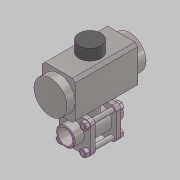
# Autodesk Inventor part: PNEUMATIC BUTT WELD BALL VALVE DN25 304L
Saved by Autodesk Inventor 2017 (Build 210142000, 142)
## iProperties
Category: Plant Design Equipment
Company: Pocket Brewery Belgium
Created: 2017-11-25
Part Number: PNEUMATIC BUTT WELD BALL VALVE DN25 304L
Material: 304L
Document SubType Name: Modeling
Designer: Demarec
Density: 8 g/cm^3
Appearance: Semi-Polished
Description: BELVEN BV3
Author: Marc Crauwels
Title: Valves
Comments: This Valve is generated with the Pocket Brewery Valve App. This software is part of the Pocket Brewery Design Suite.
Autodesk Inventor part; units mm, degrees
ref_plane "YZ Plane" through (0, 0, 0) normal (1, 0, 0) x (0, 1, 0)
ref_plane "XZ Plane" through (0, 0, 0) normal (0, 1, 0) x (-1, 0, 0)
sketch "Sketch3" plane through (0, 0, 0) normal (0, 1, 0) x (-1, 0, 0)
  line L0 (-6.4482, 15.5674) -> (6.4482, 15.5674)
  line L1 (6.4482, 15.5674) -> (15.5674, 6.4482)
  line L2 (15.5674, 6.4482) -> (15.5674, -6.4482)
  line L3 (15.5674, -6.4482) -> (6.4482, -15.5674)
  line L4 (6.4482, -15.5674) -> (-6.4482, -15.5674)
  line L5 (-6.4482, -15.5674) -> (-15.5674, -6.4482)
  line L6 (-15.5674, -6.4482) -> (-15.5674, 6.4482)
  line L7 (-15.5674, 6.4482) -> (-6.4482, 15.5674)
  circle A0 centre (0, 0) radius 16.85
  line L8 (21.375, -28.5) -> (-21.375, -28.5)
  line L9 (-28.5, -21.375) -> (-28.5, 21.375)
  line L10 (-21.375, 28.5) -> (21.375, 28.5)
  line L11 (28.5, 21.375) -> (28.5, -21.375)
  line L12 (28.5, -28.5) -> (-28.5, 28.5) construction
  line L13 (-28.5, -28.5) -> (28.5, 28.5) construction
  circle A1 centre (0, 0) radius 15.5674
  arc A2 (28.5, 21.375) -> (21.375, 28.5) centre (21.375, 21.375) ccw
  arc A3 (-21.375, 28.5) -> (-28.5, 21.375) centre (-21.375, 21.375) ccw
  arc A4 (-28.5, -21.375) -> (-21.375, -28.5) centre (-21.375, -21.375) ccw
  arc A5 (21.375, -28.5) -> (28.5, -21.375) centre (21.375, -21.375) ccw
  circle A6 centre (0, 0) radius 13.5
  circle A7 centre (21.375, 21.375) radius 4
  circle A8 centre (0, 0) radius 20.85
  dimension "oSW" = 33.7
  dimension "oFlangeW" = 57
  dimension "d2" = 7.125
  dimension "oIntDia" = 27
  dimension "oMbolt" = 8
  dimension "d16" = 4
  constraints: 28 end point, 9 tangent, 8 centre point, 8 point on circle, 8 point on line, 5 coincident, 3 equal radius, 2 horizontal, 2 midpoint, 2 parallel, 2 perpendicular, 20 other
  measures "oFlangeW" distance of L12.start L13.start
  measures "d2" radius of A2
  measures "oIntDia" diameter of A6
  measures "oMbolt" diameter of A7
extrude "Extrusion1" add sketch "Sketch3" along normal mid plane 90 contours A0 L0 | L0 A1 L7 | L7 A0 | L0 L1 A1 | A1 | A1 L6 L7 | A0 L1 | L6 A0 | L1 L2 A1 | A1 L5 L6 | A0 L2 | L5 A0 | L2 L3 A1 | A1 L4 L5 | L4 A0 | A0 L3 | L3 L4 A1
extrude "Extrusion2" add sketch "Sketch3" along normal mid plane 55 contours A0 L0 | L7 A0 | A0 L1 | L6 A0 | A0 L2 | L5 A0 | L4 A0 | A0 L3 | L8 A4 L9 A3 L10 A2 L11 A5 | A7 | A8
extrude "Extrusion3" cut sketch "Sketch3" along normal mid plane 38 contours L8 A4 L9 A3 L10 A2 L11 A5 | A7
extrude "Extrusion4" add sketch "Sketch3" along normal mid plane 70 contours A7
sketch "Sketch4" plane through (0, -27.5, 0) normal (0, -1, 0) x (1, 0, 0)
  circle A0 centre (-21.375, 21.375) radius 4 projected
  line L0 (-17.9109, 15.375) -> (-24.8391, 15.375)
  line L1 (-24.8391, 15.375) -> (-28.3032, 21.375)
  line L2 (-28.3032, 21.375) -> (-24.8391, 27.375)
  line L3 (-24.8391, 27.375) -> (-17.9109, 27.375)
  line L4 (-17.9109, 27.375) -> (-14.4468, 21.375)
  line L5 (-14.4468, 21.375) -> (-17.9109, 15.375)
  point P0 (0, 0)
  dimension "d13" = 12
  constraints: 12 end point, 1 coincident, 1 horizontal, 13 other
  measures "d13" distance between parallel lines of L0 L3
extrude "Extrusion5" add sketch "Sketch4" along normal blind 6.4
mirror "Mirror1" about plane through (0, 0, 0) normal (0, 1, 0) of "Extrusion5"
pattern_circular "Circular Pattern1" count 4 over 360 about axis through (0, 0, 0) along (0, 1, 0) of "Extrusion5", "Extrusion4", "Mirror1"
ref_plane "Work Plane1" through (0, 0, 41) normal (0, 0, 1) x (1, 0, 0)
sketch "Sketch5" plane through (0, 0, 41) normal (0, 0, 1) x (1, 0, 0)
  line L0 (-10.875, -18) -> (10.875, -18)
  line L1 (18, -10.875) -> (18, 10.875)
  line L2 (10.875, 18) -> (-10.875, 18)
  line L3 (-18, 10.875) -> (-18, -10.875)
  line L4 (-18, -18) -> (18, 18) construction
  line L5 (18, -18) -> (-18, 18) construction
  arc A0 (-18, -10.875) -> (-10.875, -18) centre (-10.875, -10.875) ccw
  arc A1 (10.875, -18) -> (18, -10.875) centre (10.875, -10.875) ccw
  arc A2 (18, 10.875) -> (10.875, 18) centre (10.875, 10.875) ccw
  arc A3 (-10.875, 18) -> (-18, 10.875) centre (-10.875, 10.875) ccw
  point P0 (0, 0)
  dimension "d21" = 36
  dimension "d22" = 7.125
  constraints: 12 end point, 8 point on circle, 8 point on line, 8 tangent, 4 centre point, 3 equal radius, 2 midpoint, 2 parallel, 2 perpendicular, 1 horizontal
  measures "d21" distance of L4.start L5.start
  measures "d22" radius of A0
extrude "Extrusion6" add sketch "Sketch5" against normal blind 7
sketch "Sketch6" plane through (0, 0, 34) normal (0, 0, -1) x (-1, 0, 0)
  circle A0 centre (0, 0) radius 13.5
  dimension "d25" = 27
  constraints: 1 centre point, 1 coincident
  measures "d25" diameter of A0
extrude "Extrusion7" add sketch "Sketch6" along normal up to surface
chamfer "Chamfer1" distance 1 angle 45 2 edges at (16.85, 45, 0) (16.85, -45, 0)
sketch "Sketch11" plane through (0, 0, 0) normal (0, 1, 0) x (-1, 0, 0)
  line L0 (30, 41) -> (-30, 41)
  line L1 (-30, 41) -> (-30, 111)
  line L2 (-30, 111) -> (30, 111)
  line L3 (30, 111) -> (30, 41)
  line L4 (-30, 111) -> (30, 41) construction
  line L5 (30, 111) -> (-30, 41) construction
  circle A0 centre (0, 76) radius 30
  line L6 (0, 111) -> (-20, 111)
  line L7 (-20, 111) -> (-20, 131)
  line L8 (-20, 131) -> (0, 131)
  line L9 (0, 131) -> (0, 111)
  circle A1 centre (0, 0) radius 20.85 projected
  line L10 (0, 0) -> (0, 76)
  line L11 (-10.875, 41) -> (10.875, 41) projected
  dimension "oCylinderWeight" = 60
  dimension "oCylinderHeight" = 70
  dimension "oCylinderDia" = 60
  dimension "d62" = 20
  dimension "d63" = 20
  constraints: 22 end point, 4 parallel, 2 horizontal, 2 midpoint, 2 perpendicular, 1 centre point, 1 collinear, 1 vertical
  measures "oCylinderWeight" distance of L1.end L2.end
  measures "oCylinderHeight" distance of L0.end L1.end
  measures "oCylinderDia" diameter of A0
  measures "d62" distance of L7.end L8.end
  measures "d63" distance of L6.end L7.end
extrude "Extrusion12" add sketch "Sketch11" along normal mid plane 144 contours A0
extrude "Extrusion13" add sketch "Sketch11" along normal mid plane 114 contours L0 L10 A0 L3 | A0 L1 L2 L3 | A0 | L0 L1 A0 L10
revolve "Revolution1" add sketch "Sketch11" angle 360 about axis through (0, 0, 131) along (0, 0, -1) contours L2 L7 L8 L9
chamfer "Chamfer3" distance 5 angle 45 4 edges at (30, 0, 111) (-30, 0, 111) (-30, 0, 41) (30, 0, 41)
equation "\"d2\" = 0.125 * oFlangeW"
equation "\"d13\" = 1.5 * oMbolt"
equation "\"d14\" = 0.8 * oMbolt"
equation "\"d22\" = d2"
equation "\"d25\" = oIntDia"
body "Solid1"
